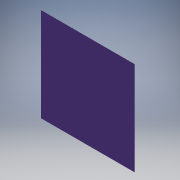
# Autodesk Inventor part: Boden
Saved by Autodesk Inventor 2018 (Build 220112000, 112)
## iProperties
Created: 2019-02-06
Part Number: Boden
Material: Generisch
Document SubType Name: Modeling
Designer: Lolob
Density: 1 g/cm^3
Appearance: Violett
Author: Lolob
Autodesk Inventor part; units mm, degrees
ref_plane "YZ Plane" through (0, 0, 0) normal (1, 0, 0) x (0, 1, 0)
ref_plane "XZ Plane" through (0, 0, 0) normal (0, 1, 0) x (-1, 0, 0)
ref_plane "XY Plane" through (0, 0, 0) normal (0, 0, 1) x (1, 0, 0)
sketch "Skizze1" plane through (0, 0, 0) normal (0, 1, 0) x (-1, 0, 0)
  line L0 (-220, 220) -> (220, 220)
  line L1 (220, 220) -> (220, -220)
  line L2 (220, -220) -> (-220, -220)
  line L3 (-220, -220) -> (-220, 220)
  line L4 (308, 0) -> (-308, 0) projected
  line L5 (0, -308) -> (0, 308) projected
  point P0 (0, 0)
  dimension "d0" = 440
  dimension "d1" = 440
  constraints: 8 end point, 2 parallel, 1 horizontal, 1 perpendicular, 2 other
  measures "d0" distance of L1.end L2.end
  measures "d1" distance of L2.end L0.start
extrude "Extrusion1" add sketch "Skizze1" along normal blind 20
chamfer "Fase1" distance 20 angle 45 4 edges at (0, 20, 220) (220, 20, 0) (0, 20, -220) (-220, 20, 0)
